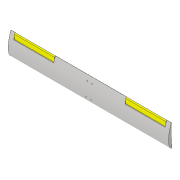
# Autodesk Inventor part: wing
Saved by Autodesk Inventor 2020 (Build 240168000, 168)
## iProperties
Created: 2019-12-24
Part Number: wing
Material: Generic
Document SubType Name: Sheet Metal
Designer: alifhabib
Density: 1 g/cm^3
Sheet Metal Rule: Default_mm
Appearance: Default
Author: alifhabib
Autodesk Inventor part; units mm, degrees
ref_plane "YZ Plane" through (0, 0, 0) normal (1, 0, 0) x (0, 1, 0)
sketch "Sketch1" plane through (0, 0, 0) normal (1, 0, 0) x (0, 1, 0)
  spline S0 degree 4 poles (287.5, 72) (275.7106, 75.6696) (272.2633, 78.0977) (241.0041, 87.3899) (212.1922, 94.1056) (186.8012, 99.4436) (162.2405, 102.6617) (136.499, 103.3609) (115.3024, 103.9082) (87.5125, 99.0497) (77.8593, 96.7101) (62.5936, 91.6603) (56.4872, 88.8369) (50.2371, 85.9481) (43.0983, 79.8721) (41.263, 78.3038) (35.0709, 71.8313) (41.0621, 66.1136) (43.5349, 66.5804) (51.0426, 65.1949) (57.2037, 65.9223) (63.437, 66.335) (78.7454, 67.9836) (88.3716, 68.7088) (116.236, 70.8678) (137.1854, 71.569) (162.8258, 72.2403) (187.1936, 73.1117) (212.5281, 72.7462) (241.0177, 72.4966) (272.1667, 71.6209) (275.8592, 71.8531) (287.5, 71.2) knots 0 0 0 0 0 0.082908 0.121264 0.162409 0.203325 0.244067 0.284728 0.322462 0.357388 0.387441 0.412707 0.436373 0.45684 0.477222 0.496964 0.514702 0.533384 0.551956 0.570848 0.593257 0.617753 0.647324 0.681959 0.719554 0.76011 0.800663 0.841217 0.881776 0.91937 1 1 1 1 1
  arc A0 (287.5, 71.2) -> (287.5, 72) centre (286.5835, 71.6) ccw
  point P0 (0, 0)
  point P1 (0, 0)
  point P2 (0, 0)
  point P3 (274.89, 76.355)
  point P4 (262.2875, 80.71)
  point P5 (237.1175, 87.97)
  point P6 (211.975, 94.0325)
  point P7 (186.8575, 99.02)
  point P8 (161.785, 102.1575)
  point P9 (136.7575, 103.3225)
  point P10 (111.775, 102.5875)
  point P11 (86.8675, 98.68)
  point P12 (74.4425, 95.465)
  point P13 (62.0425, 91.2)
  point P14 (55.855, 88.53)
  point P15 (49.685, 85.06)
  point P16 (43.5475, 80.2425)
  point P17 (40.49, 77.395)
  point P18 (37.5, 71.6)
  point P19 (40.73, 67.15)
  point P20 (43.875, 66.3)
  point P21 (50.14, 65.645)
  point P22 (56.385, 65.7925)
  point P23 (62.6225, 66.3375)
  point P24 (75.095, 67.555)
  point P25 (87.57, 68.6475)
  point P26 (112.5275, 70.43)
  point P27 (137.5025, 71.54)
  point P28 (162.485, 72.275)
  point P29 (187.47, 72.86)
  point P30 (212.4725, 72.77)
  point P31 (237.48, 72.43)
  point P32 (262.4925, 71.94)
  point P33 (274.9975, 71.7075)
  point P34 (287.5, 75)
  dimension "d0" = 1
  measures "d0" radius of A0
extrude "Plate1" add sketch "Sketch1" along normal blind 1800
ref_plane "Work Plane1" through (0, 0, 78) normal (0, 0, 1) x (1, 0, 0)
sketch "Sketch3" plane through (0, 0, 78) normal (0, 0, 1) x (1, 0, 0)
  line L0 (0, 287.5) -> (1800, 287.5) projected
  line L1 (0, 287.5) -> (50, 287.5)
  line L2 (50, 287.5) -> (500, 287.5)
  line L3 (500, 287.5) -> (500, 227.5)
  line L4 (500, 227.5) -> (50, 227.5)
  line L5 (50, 227.5) -> (50, 287.5)
  point P0 (0, 0)
  dimension "d7" = 50
  dimension "d8" = 450
  dimension "d9" = 60
  constraints: 10 end point, 2 parallel, 1 horizontal, 1 perpendicular, 1 point on line
  measures "d7" distance of L0.start L1.end
  measures "d8" distance of L3.end L4.end
  measures "d9" distance of L2.end L3.end
extrude "Extrusion1" cut sketch "Sketch3" along normal mid plane 1000
ref_plane "Work Plane2" through (900, 0, 0) normal (1, 0, 0) x (0, 0, -1)
mirror "Mirror1" about plane through (900, 0, 0) normal (1, 0, 0) of "Extrusion1"
sketch "Sketch4" plane through (0, 0, 78) normal (0, 0, 1) x (1, 0, 0)
  line L0 (500, 240.8161) -> (50, 240.8161)
  line L1 (50, 240.8161) -> (50, 376.1046)
  line L2 (50, 376.1046) -> (500, 376.1046)
  line L3 (500, 376.1046) -> (500, 240.8161)
  point P0 (0, 0)
  dimension "d12" = 450
  constraints: 8 end point, 2 parallel, 1 horizontal, 1 perpendicular
  measures "d12" distance of L1.end L2.end
extrude "Extrusion2" cut sketch "Sketch4" along normal mid plane 1000
mirror "Mirror2" about plane through (900, 0, 0) normal (1, 0, 0) of "Extrusion2"
sketch "Sketch5" plane through (1300, 227.5, 90.4191) normal (0, 1, 0) x (1, 0, 0)
  line L0 (450, 0) -> (450, 17.8321) projected
  line L1 (450, 17.8321) -> (0, 17.8321)
  line L2 (0, 17.8321) -> (0, 7.8321)
  line L3 (0, 7.8321) -> (450, 7.8321)
  line L4 (450, 7.8321) -> (450, 17.8321)
  point P0 (-1300, 90.4191)
  point P1 (450, 7.8321)
  dimension "d15" = 450
  dimension "d16" = 10
  constraints: 8 end point, 2 parallel, 1 horizontal, 1 perpendicular
  measures "d15" distance of L3.end L2.end
  measures "d16" distance of L2.end L1.end
extrude "Extrusion3" add sketch "Sketch5" along normal blind 60
mirror "Mirror3" about plane through (900, 0, 0) normal (1, 0, 0) of "Extrusion3"
fillet "Fillet1" radius 10 1 edges at (1525, 287.5, 82.587)
mirror "Mirror4" about plane through (900, 0, 0) normal (1, 0, 0) of "Fillet1"
sketch "Sketch7" plane through (0, 0, 78) normal (0, 0, 1) x (1, 0, 0)
  line L0 (500, 287.5) -> (1300, 287.5) projected
  line L1 (900, 287.5) -> (900, 163.5)
  line L2 (900, 287.5) -> (955, 287.5)
  line L3 (927.5, 287.5) -> (927.5, 237.5)
  circle A0 centre (927.5, 237.5) radius 4
  circle A1 centre (872.5, 237.5) radius 4
  line L4 (1750, 227.5) -> (1750, 240.8161) projected
  line L5 (1750, 240.8161) -> (1750, 287.5) projected
  line L6 (1750, 287.5) -> (1800, 287.5) projected
  line L7 (1800, 287.5) -> (1800, 287.5) projected
  line L8 (1750, 287.5) -> (1800, 287.5) projected
  line L9 (1750, 287.5) -> (1750, 285.643) projected
  line L10 (1750, 285.643) -> (1750, 256.2432) projected
  line L11 (1750, 256.2432) -> (1750, 240.8161) projected
  line L12 (1750, 240.8161) -> (1750, 227.5) projected
  line L13 (1750, 227.5) -> (1300, 227.5) projected
  line L14 (1300, 227.5) -> (1300, 240.8161) projected
  line L15 (1300, 240.8161) -> (1300, 256.2432) projected
  line L16 (1300, 256.2432) -> (1300, 285.643) projected
  line L17 (1300, 285.643) -> (1300, 287.5) projected
  line L18 (500, 287.5) -> (1300, 287.5) projected
  line L19 (500, 287.5) -> (500, 285.643) projected
  line L20 (500, 285.643) -> (500, 256.2432) projected
  line L21 (500, 256.2432) -> (500, 240.8161) projected
  line L22 (500, 240.8161) -> (500, 227.5) projected
  line L23 (500, 227.5) -> (50, 227.5) projected
  line L24 (50, 227.5) -> (50, 240.8161) projected
  line L25 (50, 240.8161) -> (50, 256.2432) projected
  line L26 (50, 256.2432) -> (50, 285.643) projected
  line L27 (50, 285.643) -> (50, 287.5) projected
  line L28 (0, 287.5) -> (50, 287.5) projected
  line L29 (0, 287.5) -> (0, 287.5) projected
  line L30 (0, 287.5) -> (50, 287.5) projected
  line L31 (50, 287.5) -> (50, 240.8161) projected
  line L32 (50, 240.8161) -> (50, 227.5) projected
  line L33 (50, 227.5) -> (500, 227.5) projected
  line L34 (500, 227.5) -> (500, 240.8161) projected
  line L35 (500, 240.8161) -> (500, 287.5) projected
  line L36 (500, 287.5) -> (1300, 287.5) projected
  line L37 (1300, 287.5) -> (1300, 240.8161) projected
  line L38 (1300, 240.8161) -> (1300, 227.5) projected
  line L39 (1300, 227.5) -> (1750, 227.5) projected
  line L40 (927.5, 287.5) -> (927.5, 87.5)
  circle A2 centre (927.5, 87.5) radius 4
  circle A3 centre (872.5, 237.5) radius 4
  circle A4 centre (872.5, 87.5) radius 4
  point P0 (0, 0)
  dimension "d31" = 124
  dimension "d32" = 55
  dimension "d33" = 50
  dimension "d34" = 8
  dimension "d35" = 200
  dimension "d36" = 8
  constraints: 8 end point, 5 centre point, 5 symmetric about line, 4 coincident, 2 midpoint, 2 point on line, 2 vertical, 3 other
  measures "d31" distance of L1.start L1.end
  measures "d32" distance of L1.start L2.end
  measures "d33" distance of L3.start L3.end
  measures "d34" diameter of A0
  measures "d35" distance of L3.start L40.end
  measures "d36" diameter of A2
extrude "Extrusion5" cut sketch "Sketch7" along normal mid plane 6000
equation "\"d1\" = Thickness"
equation "\"Thickness\" = 1800"
body "Solid1"
